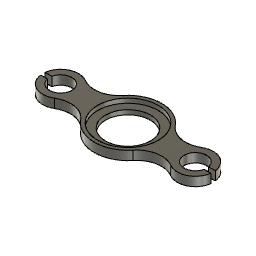
Model 12 (Autodesk Fusion 360 design; units mm, degrees)
Autodesk Fusion 360 part; units mm, degrees
sketch "Sketch2" plane through (0, 0, 0) normal (0, 0, 1) x (1, 0, 0)
  circle A0 centre (0, 0) radius 50
  circle A1 centre (0, 0) radius 67.5
  line L0 (0, 0) -> (150, 0) construction
  line L1 (0, 0) -> (-150, 0) construction
  line L2 (-150, 0) -> (-150, 5) construction
  line L3 (-150, 0) -> (-150, -5) construction
  line L4 (-174.4949, 5) -> (-189.6863, 5)
  line L5 (-174.4949, -5) -> (-189.6863, -5)
  line L6 (150, 0) -> (150, 5) construction
  line L7 (150, 0) -> (150, -5) construction
  line L8 (174.4949, 5) -> (189.6863, 5)
  line L9 (174.4949, -5) -> (189.6863, -5)
  arc A2 (-174.4949, -5) -> (-174.4949, 5) centre (-150, 0) ccw
  arc A3 (174.4949, 5) -> (174.4949, -5) centre (150, 0) ccw
  arc A4 (-129.4737, 34.3318) -> (-58.4135, 47.0411) centre (-101.25, 81.538) ccw
  arc A5 (-58.4135, -47.0411) -> (-129.4737, -34.3318) centre (-101.25, -81.538) ccw
  arc A6 (129.4737, -34.3318) -> (58.4135, -47.0411) centre (101.25, -81.538) ccw
  arc A7 (58.4135, 47.0411) -> (129.4737, 34.3318) centre (101.25, 81.538) ccw
  arc A8 (-189.6863, -5) -> (-129.4737, -34.3318) centre (-150, 0) ccw
  arc A9 (-129.4737, 34.3318) -> (-189.6863, 5) centre (-150, 0) ccw
  arc A10 (189.6863, 5) -> (129.4737, 34.3318) centre (150, 0) ccw
  arc A11 (129.4737, -34.3318) -> (189.6863, -5) centre (150, 0) ccw
  arc A12 (-58.4135, -47.0411) -> (58.4135, -47.0411) centre (0, 0) ccw
  arc A13 (58.4135, 47.0411) -> (-58.4135, 47.0411) centre (0, 0) ccw
  dimension "d13" = 100
  dimension "d14" = 135
  dimension "d15" = 150
  dimension "d16" = 150
  dimension "d17" = 150
  dimension "d18" = 50
  dimension "d19" = 80
  dimension "d20" = 50
  dimension "d21" = 80
  dimension "d22" = 5
  dimension "d23" = 5
  dimension "d24" = 5
  dimension "d25" = 5
  dimension "d26" = 110
  dimension "d27" = 110
  dimension "d28" = 110
  dimension "d30" = 110
  constraint coincident A0.centre A1.centre
  constraint concentric A1 A12
  constraint horizontal L0
  constraint horizontal L1
  constraint coincident L1.end L2.start
  constraint concentric A2 A8
  constraint coincident L0.end L6.start
  constraint concentric A3 A10
  constraint perpendicular L1 L2
  constraint perpendicular L1 L3
  constraint perpendicular L2 L4
  constraint perpendicular L3 L5
  constraint perpendicular L0 L6
  constraint perpendicular L0 L7
  constraint perpendicular L6 L8
  constraint perpendicular L7 L9
  constraint tangent A4 A12
  constraint tangent A4 A8
  constraint coincident A4.start A8
  constraint tangent A5 A12
  constraint tangent A5 A8
  constraint tangent A7 A12
  constraint tangent A7 A10
  constraint tangent A6 A12
  constraint tangent A6 A10
  constraint coincident A6.start A10
  constraint coincident A7.start A12
  constraint concentric A8 A9
  constraint concentric A10 A11
  constraint concentric A12 A13
  measures "d13" diameter of A0
  measures "d14" diameter of A1
  measures "d15" diameter of A12
  measures "d16" distance of A0.centre L0.end
  measures "d17" distance of A0.centre L1.end
  measures "d18" diameter of A2
  measures "d19" diameter of A8
  measures "d20" diameter of A3
  measures "d21" diameter of A10
  measures "d22" distance of L1.end L2.end
  measures "d23" distance of L1.end L3.end
  measures "d24" distance of L0.end L6.end
  measures "d25" distance of L0.end L7.end
  measures "d26" diameter of A4
  measures "d27" diameter of A5
  measures "d28" diameter of A6
  measures "d30" diameter of A7
extrude "Extrude2" add sketch "Sketch2" along normal blind 10 contours A1
extrude "Extrude3" add sketch "Sketch2" along normal blind 20 contours L4 L5 L8 L9 A2 A3 A4 A5 A6 A7 A8 A9 A10 A11 A12 A13
